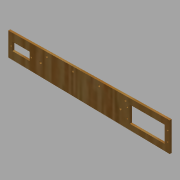
# Autodesk Inventor part: segment2a
Saved by Autodesk Inventor 2013 (Build 170138000, 138)
## iProperties
Created: 2014-10-09
Part Number: segment2a
Material: Plywood, Finish
Document SubType Name: Modeling
Designer: Masta
Density: 0.552 g/cm^3
Mass: 27.6958 g
Surface Area: 217.441 cm^2
Volume: 50.1735 cm^3
Author: Masta
Autodesk Inventor part; units mm, degrees
ref_plane "YZ Plane" through (0, 0, 0) normal (1, 0, 0) x (0, 1, 0)
ref_plane "XZ Plane" through (0, 0, 0) normal (0, 1, 0) x (-1, 0, 0)
ref_plane "XY Plane" through (0, 0, 0) normal (0, 0, 1) x (1, 0, 0)
sketch "Sketch1" plane through (0, 0, 0) normal (0, 1, 0) x (-1, 0, 0)
  line L0 (0, 0) -> (45.5, 0)
  line L1 (217, -7) -> (247, -7)
  line L2 (247, -7) -> (247, 7)
  line L3 (247, 7) -> (217, 7)
  line L4 (217, 7) -> (217, -7)
  line L5 (217, -7) -> (247, 7) construction
  line L6 (247, -7) -> (217, 7) construction
  line L7 (232, 0) -> (246.5, 0) construction
  line L8 (0, 0) -> (18.5, 0) construction
  line L9 (217, 0) -> (240, 0) construction
  line L10 (0, 0) -> (-14.5, 0)
  line L11 (-23, 0) -> (-23, 25)
  line L12 (-23, 25) -> (254, 20)
  line L13 (254, 20) -> (254, 0)
  line L14 (254, 0) -> (240, 0) construction
  line L15 (254, 0) -> (247, 0)
  line L16 (-14.5, 14.25) -> (45.5, 14.25)
  line L17 (45.5, 14.25) -> (45.5, -14.25)
  line L18 (45.5, -14.25) -> (-14.5, -14.25)
  line L19 (-14.5, -14.25) -> (-14.5, 14.25)
  line L20 (-14.5, 14.25) -> (45.5, -14.25) construction
  line L21 (45.5, 14.25) -> (-14.5, -14.25) construction
  line L22 (-19, 8.5) -> (50, 8.5) construction
  line L23 (50, 8.5) -> (50, -8.5) construction
  line L24 (50, -8.5) -> (-19, -8.5) construction
  line L25 (-19, -8.5) -> (-19, 8.5) construction
  line L26 (-19, 8.5) -> (50, -8.5) construction
  line L27 (50, 8.5) -> (-19, -8.5) construction
  line L28 (45.5, 0) -> (217, 0)
  line L29 (-14.5, 0) -> (-23, 0)
  line L30 (-23, 0) -> (0, 0) construction
  line L31 (249.5, 2.5) -> (214.5, 2.5) construction
  line L32 (214.5, 2.5) -> (214.5, -2.5) construction
  line L33 (214.5, -2.5) -> (249.5, -2.5) construction
  line L34 (249.5, -2.5) -> (249.5, 2.5) construction
  line L35 (249.5, 2.5) -> (214.5, -2.5) construction
  line L36 (214.5, 2.5) -> (249.5, -2.5) construction
  point P0 (15.5, 0)
  point P1 (15.5, 0)
  point P2 (62, 0)
  point P3 (199, 0)
  point P4 (53.3745, 16.6203)
  point P5 (214.5, 0)
  point P6 (249.5, 0)
  dimension "d21" = 240
  dimension "d22" = 30
  dimension "d23" = 14
  dimension "d24" = 7
  dimension "d25" = 14.5
  dimension "d28" = 18.5
  dimension "d37" = 20
  dimension "d38" = 25
  dimension "d39" = 60
  dimension "d40" = 28.5
  dimension "d41" = 69
  dimension "d42" = 17
  dimension "d43" = 14.5
  dimension "d52" = 7
  dimension "d53" = 4
  dimension "d54" = 85
  dimension "d55" = 35
  dimension "d56" = 5
  dimension "d57" = 55
  dimension "d65" = 7
  dimension "d76" = 14
  dimension "d77" = 277
  dimension "d78" = 23
  constraints: 74 end point, 16 midpoint, 9 parallel, 8 perpendicular, 7 horizontal, 6 point on line, 4 coincident, 3 collinear
  measures "d21" distance of L0.start L9.end
  measures "d22" distance of L3.end L2.end
  measures "d23" distance of L2.end L1.end
  measures "d24" distance from line of L9.end L2
  measures "d25" distance of L7.start L7.end
  measures "d28" distance of L0.start L8.end
  measures "d37" distance of L12.end L13.end
  measures "d38" distance of L11.start L11.end
  measures "d39" distance of L17.end L18.end
  measures "d40" distance of L16.end L17.end
  measures "d41" distance of L23.end L24.end
  measures "d42" distance of L22.end L23.end
  measures "d43" distance from line of L19 point (0, 0)
  measures "d52" distance between parallel lines of L13 L2
  measures "d53" distance between parallel lines of L25 L11
  measures "d54" distance from line of L11 point (62, 0)
  measures "d55" distance of L32.end L33.end
  measures "d56" distance of L31.end L32.end
  measures "d57" distance from line of L13 point (199, 0)
  measures "d65" distance from line of L12 point (53.375, 16.62)
  measures "d76" distance from line of L13 L9.end
  measures "d77" distance between parallel lines of L13 L11
  measures "d78" distance from line of L11 point (0, 0)
extrude "Extrusion1" add sketch "Sketch1" along normal blind 3.5 contours L17 L16 L19 L29 L11 L12 L13 L15 L2 L3 L4 L28
hole "Hole3" at (0, 0, 0) at (19, 0, 8.5) at (-50, 0, 8.5) at (-214.5, 0, 0) at (-249.5, 0, 0) direction (0, 1, 0) diameter 3 end through all
fillet "Fillet1" [suppressed]
mirror "Mirror1" about plane through (-45.5, 0, 0) normal (0, 0, -1)
hole "Hole4" at (-62, 0, 0) at (-199, 0, 0) direction (0, 1, 0) diameter 4.5 end through all
hole "Hole5" at (-53.3745, 0, 16.6203) direction (0, 1, 0) diameter 4 end through all
pattern_linear "Rectangular Pattern1" count 4 spacing 45 along (-0.9998371, 0, -0.0180476) of "Hole5"
body "Solid1"
